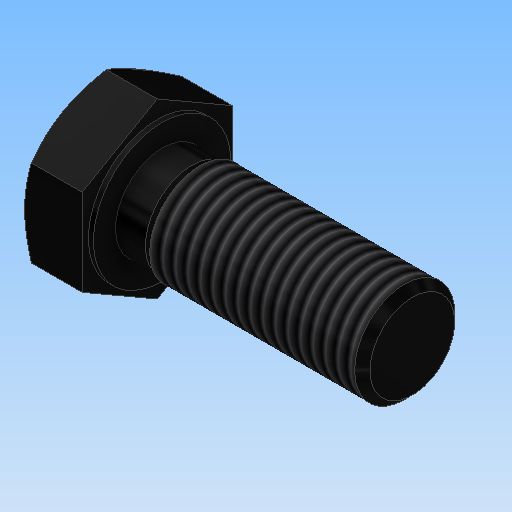
# Autodesk Inventor part: DIN 933 - M16  x 40
Saved by Autodesk Inventor 2020.1 (Build 241239000, 239)
## iProperties
Comments: To add or edit properties for Autodesk Inventor files, use iProperties.
Shininess: 64.0
Length Units: 11269
Angle Units: 11279
Time Units: 11290
Mass Units: 11283
Length Display Precision: 3
Angle Display Precision: 2
Compacted: True
Alert: To add or edit properties for Autodesk Inventor files, use iProperties.
Library Location: C:\ap\Inventor 6\content
Library: local
SubLibrary: DIN
Family: 19
Member: 282
Member Major Revision: 1
Member Minor Revision: 1
Created: 2003-02-27
Part Number: DIN 933 - M16  x 40
Vendor: Autodesk Inc.
Document SubType Name: Modeling
Designer: Joe M
Description: Sechskantschraube
Standard: DIN 933 M16  x 40
Engineer: Joe M
Material: Generic
Density: 1 g/cm^3
Appearance: Glossy - Black
Density: 0.0
Volumn: 0.0
Area: 0.0
PropertySet Name: Model Information
Control State: 0
Master: False
Checked Out: False
Author: Joe M
Autodesk Inventor part; units mm, degrees
ref_plane "YZ Plane" through (0, 0, 0) normal (1, 0, 0) x (0, 1, 0)
ref_plane "XZ Plane" through (0, 0, 0) normal (0, 1, 0) x (-1, 0, 0)
ref_plane "XY Plane" through (0, 0, 0) normal (0, 0, 1) x (1, 0, 0)
sketch "Skizze1" plane through (0, 0, 0) normal (0, 0, 1) x (1, 0, 0)
  line L0 (0, 11) -> (0, 7.4587)
  line L1 (6, 8) -> (40, 8)
  line L2 (40, 8) -> (40, 0)
  line L3 (40, 0) -> (-0.8001, 0)
  line L4 (-4.8801, 0) -> (52.24, 0) projected
  line L5 (-0.8001, 0) -> (-0.8001, 11)
  line L6 (-0.8001, 11) -> (0, 11)
  line L7 (6, 8) -> (4.773, 7.4587)
  line L8 (4.773, 7.4587) -> (0, 7.4587)
  line L9 (0, -1.1) -> (0, 14.3) projected
  dimension "d0" = 40
  dimension "d1" = 34
  dimension "d2" = 16
  dimension "d9" = 0.8001
  dimension "d10" = 22
  dimension "d13" = 1.227
  dimension "d14" = 14.9175
  constraints: 16 end point, 2 collinear, 2 perpendicular, 1 parallel
  measures "d0" distance between parallel lines of L2 L0
  measures "d1" distance from line of L1.start L2
  measures "d2" diameter of L1 L3
  measures "d9" distance between parallel lines of L5 L0
  measures "d10" diameter of L6 L3
  measures "d13" horizontal distance of L1.start L7.end
  measures "d14" diameter of L8 L3
revolve "Körper" add sketch "Skizze1" angle 360 about axis through (40, 0, 0) along (-1, 0, 0)
sketch "Skizze2" plane through (-0.8001, 0, 0) normal (-1, 0, 0) x (0, 0, 1)
  line L0 (0, 13.8564) -> (12, 6.9282)
  line L1 (12, 6.9282) -> (12, -6.9282)
  line L2 (12, -6.9282) -> (0, -13.8564)
  line L3 (0, -13.8564) -> (-12, -6.9282)
  line L4 (-12, -6.9282) -> (-12, 6.9282)
  line L5 (-12, 6.9282) -> (0, 13.8564)
  point P0 (0, 0)
  point P1 (0, 0)
  dimension "d11" = 24
  constraints: 12 end point, 1 coincident, 1 vertical, 11 other
  measures "d11" distance between parallel lines of L4 L1
extrude "Kopf" add sketch "Skizze2" along normal blind 9.2
sketch "Skizze4" plane through (0, 0, 0) normal (0, 0, 1) x (1, 0, 0)
  line L0 (-10.0001, 12) -> (-10.0001, 13.8564)
  line L1 (-10.0001, 13.8564) -> (-8.9283, 13.8564)
  line L2 (-8.9283, 13.8564) -> (-10.0001, 12)
  line L3 (-10.9201, 0) -> (1.9599, 0) projected
  line L4 (-0.8001, 13.8564) -> (-10.0001, 13.8564) projected
  line L5 (-10.0001, 6.9282) -> (-10.0001, 13.8564) projected
  dimension "d5" = 30
  dimension "d19" = 24
  constraints: 6 end point, 2 collinear, 1 perpendicular, 1 vertical
  measures "d5" angle of L2 L0
  measures "d19" diameter of L0.start L3
revolve "Fase1" cut sketch "Skizze4" angle 360 about axis through (-10, 0, 0) along (1, 0, 0)
thread "Gewinde" size "M16x2" class "6g" standard "ANSI Metric M Profile" length 34
chamfer "Fase2" distance 1.2269 distance2 1.227 1 edges at (40, -8, 0) measured on face at (40, -0.1598, 1.3157)
equation "\"d0\" = NLG"
equation "\"d1\" = GEL"
equation "\"d2\" = GD"
equation "\"d10\" = SD2"
equation "\"d14\" = BDM"
equation "\"d11\" = SW"
equation "\"d3\" = KOH - SD"
equation "\"d5\" = ANG1"
equation "\"d19\" = SW0"
equation "\"d15\" = GEL"
equation "\"d6\" = -0.5 * SPD + 0.5 * GD"
equation "\"NLG\" = 40"
equation "\"GD\" = NND"
equation "\"BDM\" = 14.91747"
equation "\"KOH\" = 10"
equation "\"GEL\" = 34"
equation "\"SW\" = 24"
equation "\"SW0\" = 24"
equation "\"SPD\" = NND - 1.2269 * TPU"
equation "\"SD2\" = 22"
equation "\"SD\" = 0.8"
equation "\"ANG1\" = 30deg"
equation "\"GAL\" = 0.61345 * TPU"
equation "\"GUL\" = 0.61345 * TPU"
equation "\"RR\" = 0.6"
equation "\"TOA\" = 30deg"
equation "\"PTC\" = TPU"
equation "\"GD1\" = THREADDIA - 1.2269 * TPU"
equation "\"TPU\" = 2"
equation "\"THREADDIA\" = 16"
equation "\"E0\" = 1.155 * SW"
equation "\"NND\" = 16"
body "Solid1"
